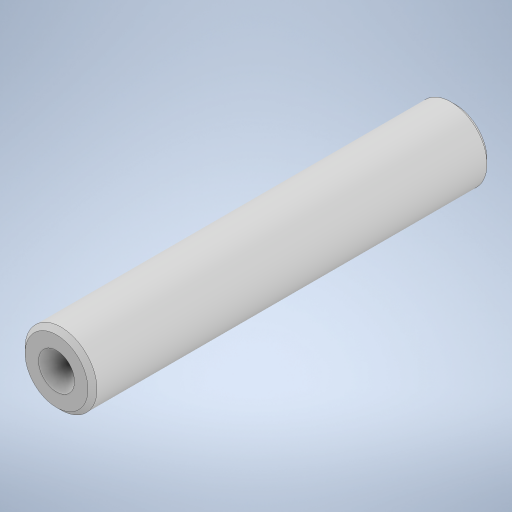
# Autodesk Inventor part: MotorBeltTensionerAxis
Saved by Autodesk Inventor 2023 (Build 270158000, 158)
## iProperties
Created: 2022-01-06
Part Number: MotorBeltTensionerAxis
Material: Generic
Document SubType Name: Modeling
Designer: Jochen
Density: 1 g/cm^3
Appearance: Default
Author: Jochen
Autodesk Inventor part; units mm, degrees
ref_plane "YZ Plane" through (0, 0, 0) normal (1, 0, 0) x (0, 1, 0)
ref_plane "XZ Plane" through (0, 0, 0) normal (0, 1, 0) x (-1, 0, 0)
ref_plane "XY Plane" through (0, 0, 0) normal (0, 0, 1) x (1, 0, 0)
sketch "Sketch1" plane through (0, 0, 0) normal (0, 0, 1) x (1, 0, 0)
  circle A0 centre (0, 0) radius 2
  dimension "d0" = 4
  constraints: 1 centre point, 1 coincident
  measures "d0" diameter of A0
extrude "Extrusion1" add sketch "Sketch1" along normal blind 22.2
chamfer "Chamfer1" distance 0.25 angle 45 2 edges at (-2, 0, 22.2) (-2, 0, 0)
sketch "Sketch2" plane through (0, 0, 0) normal (1, 0, 0) x (0, 1, 0)
  line L0 (2, 0.25) -> (1.75, 0) projected
  line L1 (1.75, 0) -> (-1.75, 0) projected
  line L2 (-1.75, 0) -> (-2, 0.25) projected
  line L3 (-2, 0.25) -> (-2, 21.95) projected
  line L4 (-2, 21.95) -> (-1.75, 22.2) projected
  line L5 (-1.75, 22.2) -> (1.75, 22.2) projected
  line L6 (1.75, 22.2) -> (2, 21.95) projected
  line L7 (2, 21.95) -> (2, 0.25) projected
  line L8 (-1.75, 22.2) -> (1.75, 22.2) projected
  line L9 (1, 22.2) -> (0, 21.2)
  line L10 (0, 21.2) -> (0, 22.2)
  line L11 (1, 0) -> (0, 1)
  line L12 (0, 1) -> (0, 0)
  line L13 (0, -4.4) -> (0, 26.4) projected
  dimension "d6" = 1
  dimension "d7" = 1
  dimension "d8" = 45
  constraints: 8 end point, 3 midpoint, 2 collinear, 2 point on line
  measures "d6" distance of point (0, 22.2) L9.start
  measures "d7" distance of point (0, 0) L11.start
  measures "d8" angle of L9 L10
revolve "Revolution1" cut sketch "Sketch2" angle 360 about axis through (0, 0, -10) along (0, 0, 1) contours L1 L12 L11 | L9 L10 L5
equation "\"d7\" = d6"
body "Solid1"
